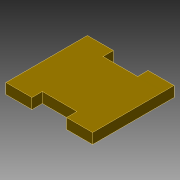
# Autodesk Inventor part: Стойка_В5
Saved by Autodesk Inventor 2021.3 (Build 253353000, 353)
## iProperties
RuleStatus: InUse
Part Number: Стойка_В5
Checked By: Якушев
Engr Approved By: Малов
Material: По умолчанию1
Document SubType Name: Modeling
Mfg Approved By: Судаков
Designer: Смирнов
Density: 1 g/cm^3
Appearance: Золото
AfterMaterialChange0: Материал
BeforeDocSave0: Материал
AfterAnyiPropertyChange0: Материал
Материал: По умолчанию1
Author: Смирнов
Autodesk Inventor part; units mm, degrees
ref_plane "YZ Plane" through (0, 0, 0) normal (1, 0, 0) x (0, 1, 0)
ref_plane "XZ Plane" through (0, 0, 0) normal (0, 1, 0) x (-1, 0, 0)
ref_plane "XY Plane" through (0, 0, 0) normal (0, 0, 1) x (1, 0, 0)
sketch "Эскиз1" plane through (0, 0, 0) normal (0, 0, 1) x (1, 0, 0)
  line L0 (25, -17.5) -> (-25, -17.5)
  line L1 (-25, -17.5) -> (-25, 17.5)
  line L2 (-25, 17.5) -> (25, 17.5)
  line L3 (25, 17.5) -> (25, -17.5)
  line L4 (25, -17.5) -> (-25, 17.5) construction
  line L5 (-25, -17.5) -> (25, 17.5) construction
  line L6 (-25, 17.5) -> (-10, 17.5)
  line L7 (-10, 17.5) -> (-10, 23.5)
  line L8 (-10, 23.5) -> (-25, 23.5)
  line L9 (-25, 23.5) -> (-25, 17.5)
  line L10 (25, 17.5) -> (10, 17.5)
  line L11 (10, 17.5) -> (10, 23.5)
  line L12 (10, 23.5) -> (25, 23.5)
  line L13 (25, 23.5) -> (25, 17.5)
  line L14 (-25, -17.5) -> (-10, -17.5)
  line L15 (-10, -17.5) -> (-10, -23.5)
  line L16 (-10, -23.5) -> (-25, -23.5)
  line L17 (-25, -23.5) -> (-25, -17.5)
  line L18 (25, -17.5) -> (10, -17.5)
  line L19 (10, -17.5) -> (10, -23.5)
  line L20 (10, -23.5) -> (25, -23.5)
  line L21 (25, -23.5) -> (25, -17.5)
  line L22 (0, 0) -> (0, 45.655) construction
  point P0 (-10, -17.5)
  point P1 (10, 17.5)
  dimension "d0" = 50
  dimension "d1" = 35
  dimension "d2" = 6
  dimension "d3" = 15
  constraints: 46 end point, 10 parallel, 5 horizontal, 5 perpendicular, 4 point on line, 2 midpoint, 1 collinear, 1 vertical, 1 other
  measures "d0" distance of L1.end L2.end
  measures "d1" distance of L2.end L0.start
  measures "d2" distance of L10.end L11.end
  measures "d3" distance of L11.end L12.end
extrude "Выдавливание1" add sketch "Эскиз1" along normal mid plane 6
